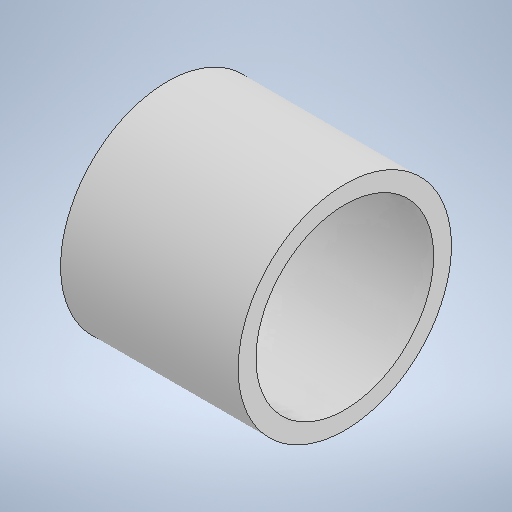
# Autodesk Inventor part: Distanzhülse
Saved by Autodesk Inventor 2025 (Build 290162010, 162A)
## iProperties
Created: 2024-11-15
Part Number: Distanzhülse
Material: Generisch
Document SubType Name: Modeling
Designer: jensb
Density: 1 g/cm^3
Appearance: Vorgabe
Author: jensb
Autodesk Inventor part; units mm, degrees
ref_plane "YZ Plane" through (0, 0, 0) normal (1, 0, 0) x (0, 1, 0)
ref_plane "XZ Plane" through (0, 0, 0) normal (0, 1, 0) x (-1, 0, 0)
ref_plane "XY Plane" through (0, 0, 0) normal (0, 0, 1) x (1, 0, 0)
sketch "Skizze1" plane through (0, 0, 0) normal (0, 0, 1) x (1, 0, 0)
  line L0 (-23.5268, 11.0714) -> (30.4911, 11.0714)
  line L1 (-21.5018, 16.0714) -> (-11.5018, 16.0714)
  line L2 (-21.5018, 16.0714) -> (-21.5018, 17.0714)
  line L3 (-11.5018, 16.0714) -> (-11.5018, 17.0714)
  line L4 (-21.5018, 17.0714) -> (-11.5018, 17.0714)
  point P0 (0, 0)
  dimension "d0" = 10
  dimension "d1" = 10
  dimension "d2" = 12
  constraints: 10 end point, 2 horizontal, 2 vertical, 1 perpendicular
  measures "d0" diameter of L1 L0
  measures "d1" distance of L1.start L1.end
  measures "d2" diameter of L4 L0
revolve "Umdrehung1" add sketch "Skizze1" angle 360 about axis through (-23.5268, 11.0714, 0) along (1, 0, 0)
